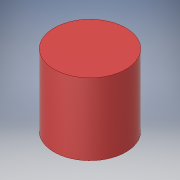
# Autodesk Inventor part: Cylindre
Saved by Autodesk Inventor 2019.3 (Build 233278000, 278)
## iProperties
Created: 2019-03-04
Part Number: Cylindre
Material: Plastique ABS
Document SubType Name: Modeling
Designer: Houba Guillaume
Mass: 53.2814 g
Surface Area: 75.3982 cm^2
Volume: 50.2655 cm^3
Density: 1.06 g/cm^3
Appearance: Lisse - Rouge
Author: Houba Guillaume
## iProperties of the stored document Cylindre_Impression 3D.ipt
Created: 2019-03-04
Part Number: Cylindre_Impression 3D
Material: Générique
Document SubType Name: Modeling
Designer: Houba Guillaume
Mass: 50.2655 g
Surface Area: 75.3982 cm^2
Volume: 50.2655 cm^3
Density: 1 g/cm^3
Appearance: Par défaut
Author: Houba Guillaume
Autodesk Inventor part; units mm, degrees
ref_plane "YZ Plane" through (0, 0, 0) normal (1, 0, 0) x (0, 1, 0)
ref_plane "XZ Plane" through (0, 0, 0) normal (0, 1, 0) x (-1, 0, 0)
ref_plane "XY Plane" through (0, 0, 0) normal (0, 0, 1) x (1, 0, 0)
sketch "Esquisse1" plane through (0, 0, 0) normal (0, 1, 0) x (-1, 0, 0)
  circle A0 centre (0, 0) radius 20
  dimension "d0" = 40
  constraints: 1 centre point
  measures "d0" diameter of A0
extrude "Cylindre1" add sketch "Esquisse1" along normal blind 40
equation "\"d0\" = dd1"
equation "\"d1\" = dd0"
equation "\"dd0\" = 40"
equation "\"dd1\" = 40"
